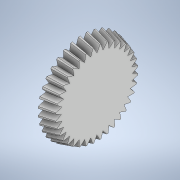
# Autodesk Inventor part: motor driven gear
Saved by Autodesk Inventor 2022 (Build 260153000, 153)
## iProperties
Created: 2021-11-09
Part Number: motor driven gear
Material: Generic
Document SubType Name: Modeling
Designer: a-dubs
Density: 1 g/cm^3
Appearance: Default
Author: a-dubs
Autodesk Inventor part; units mm, degrees
ref_plane "YZ Plane" through (0, 0, 0) normal (1, 0, 0) x (0, 1, 0)
ref_plane "XZ Plane" through (0, 0, 0) normal (0, 1, 0) x (-1, 0, 0)
ref_plane "XY Plane" through (0, 0, 0) normal (0, 0, 1) x (1, 0, 0)
sketch "Sketch1" plane through (0, 0, 0) normal (0, 1, 0) x (-1, 0, 0)
  line L0 (0, 0) -> (0, 18)
  line L1 (0, 18) -> (7, 18)
  line L2 (7, 18) -> (7, 0)
  line L3 (7, 0) -> (0, 0)
  line L4 (0, 18) -> (0, 21)
  line L5 (7, 18) -> (7, 20)
  line L6 (7, 20) -> (0, 18)
  line L7 (0, 21) -> (7, 23)
  line L8 (7, 23) -> (7, 20)
  dimension "d0" = 18
  dimension "d1" = 7
  dimension "d2" = 3
  dimension "d3" = 2
  constraints: 18 end point, 3 perpendicular, 2 point on line, 2 vertical, 1 collinear, 1 parallel
  measures "d0" distance of L0.start L0.end
  measures "d1" distance of L0.end L1.end
  measures "d2" distance of L0.end L4.end
  measures "d3" distance of L1.end L5.end
revolve "Revolution1" add sketch "Sketch1" angle 360 about axis through (-7, 0, 0) along (1, 0, 0) contours L0 L1 L2 L3 | L6 L5 L1
revolve "Revolution2" add sketch "Sketch1" angle 10 about axis through (-7, 0, 0) along (-1, 0, 0) contours L4 L7 L8 L6
chamfer "Chamfer1" distance 2.75 angle 30 1 edges at (-3.5, 3.8203, 21.6658) measured on face at (-3.6374, 3.7368, 21.1923)
chamfer "Chamfer2" distance 2.75 angle 30 1 edges at (-3.5, 0, 22) measured on face at (-3.6374, 0, 21.5192)
pattern_circular "Circular Pattern1" count 36 over 360 about axis through (-3.5, 0, 0) along (-1, 0, 0)
body "Solid1"
